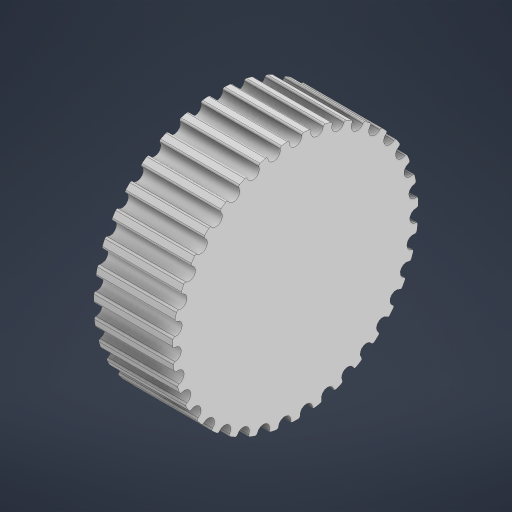
# Autodesk Inventor part: GT2 Pulley
Saved by Autodesk Inventor 2024 (Build 280153000, 153)
## iProperties
Created: 2023-10-25
Part Number: GT2 Pulley
Material: Generic
Document SubType Name: Modeling
Designer: avsar
Density: 1 g/cm^3
Appearance: Default
Author: avsar
Autodesk Inventor part; units mm, degrees
ref_plane "YZ Plane" through (0, 0, 0) normal (1, 0, 0) x (0, 1, 0)
ref_plane "XZ Plane" through (0, 0, 0) normal (0, 1, 0) x (-1, 0, 0)
ref_plane "XY Plane" through (0, 0, 0) normal (0, 0, 1) x (1, 0, 0)
sketch "Sketch1" plane through (0, 0, 0) normal (1, 0, 0) x (0, 1, 0)
  circle A0 centre (0, 0) radius 10.8868 construction
  circle A1 centre (0, 0) radius 10.1368 construction
  line L0 (0, 0) -> (10.8868, 0) construction
  line L1 (0, 0) -> (0, -10.8868) construction
  circle A2 centre (10.6918, 0) radius 0.555 construction
  line L2 (0, 0) -> (10.7119, -1.9439) construction
  circle A3 centre (10.52, -1.9091) radius 0.555 construction
  circle A4 centre (10.7137, -0.7047) radius 0.15 construction
  circle A5 centre (10.6673, -1.2197) radius 0.15 construction
  arc A6 (10.1368, 0) -> (10.709, -0.5547) centre (10.6918, 0) ccw
  arc A7 (10.8634, -0.7145) -> (10.709, -0.5547) centre (10.7137, -0.7047) ccw
  arc A8 (10.8164, -1.2367) -> (10.8634, -0.7145) centre (0, 0) ccw
  arc A9 (10.636, -1.3664) -> (10.8164, -1.2367) centre (10.6673, -1.2197) ccw
  arc A10 (10.636, -1.3664) -> (9.9739, -1.81) centre (10.52, -1.9091) ccw
  arc A11 (9.9739, -1.81) -> (10.1368, 0) centre (0, 0) ccw
  dimension "d0" = 21.7737
  dimension "d1" = -0.75
  dimension "d2" = 1.11
  dimension "d4" = 79.714
  dimension "d5" = 0.3
  constraints: 25 point on circle, 12 centre point, 8 equal radius, 8 tangent, 6 end point, 4 point on line, 1 coincident, 1 concentric, 1 horizontal, 1 perpendicular
  measures "d0" diameter of A0
  measures "d1" radial gap between concentric circles of A0 A1
  measures "d2" diameter of A2
  measures "d4" angle of L1 L2
  measures "d5" diameter of A4
extrude "Extrusion1" add sketch "Sketch1" along normal mid plane 7
pattern_circular "Circular Pattern1" count 35 over 360 about axis through (-10, 0, 0) along (1, 0, 0) of "Extrusion1"
sketch "Sketch2" plane through (0, 0, 0) normal (1, 0, 0) x (0, 1, 0)
  arc A0 (9.9739, 1.81) -> (10.636, 1.3664) centre (10.52, 1.9091) ccw projected
  circle A1 centre (0, 0) radius 10.1368
  constraints: 1 coincident, 3 other
extrude "Extrusion2" add sketch "Sketch2" along normal mid plane 7
equation "\"d0\" = OD_"
equation "\"d1\" = H_"
equation "\"d2\" = BTD_"
equation "\"d4\" = TH_"
equation "\"d5\" = PTR_"
equation "\"d6\" = EX_"
equation "\"d11\" = EX_"
equation "\"U_\" = 0.254"
equation "\"H_\" = -0.75"
equation "\"P_\" = 2"
equation "\"BTD_\" = 1.11"
equation "\"PTR_\" = 0.3"
equation "\"EX_\" = 7"
equation "\"OD_\" = PD_ - 2 * U_"
equation "\"TH_\" = 79.714286deg"
equation "\"PD_\" = 22.281692"
body "Solid1"
